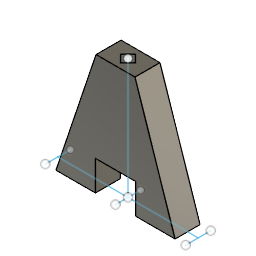
Leg (Autodesk Fusion 360 design; units mm, degrees)
part number: 2025-11-29-20-59-17-478
Autodesk Fusion 360 part; units mm, degrees
sketch "Sketch1" plane through (0, 0, 0) normal (0, 0, 1) x (1, 0, 0)
sketch "Sketch2" plane through (0, 0, 0) normal (0, 0, 1) x (1, 0, 0)
  circle A0 centre (0, 0) radius 100
  constraint coincident A0.centre origin
sketch "Sketch3" plane through (0, 0, 0) normal (0, 0, 1) x (1, 0, 0)
  circle A0 centre (0, -70) radius 17.5
  circle A1 centre (0, 70) radius 17.5
  dimension "d3" = 35
  dimension "d4" = 35
  measures "d3" diameter of A0
  measures "d4" diameter of A1
sketch "Sketch4" plane through (0, 0, 0) normal (0, 0, 1) x (1, 0, 0)
  circle A0 centre (0, -70) radius 5.25
  circle A1 centre (0, 70) radius 5.25
  dimension "d7" = 10.5
  dimension "d8" = 10.5
  measures "d7" diameter of A0
  measures "d8" diameter of A1
sketch "Sketch5" plane through (0, 0, 30) normal (0, 0, 1) x (-1, 0, 0)
  circle A0 centre (0, -70) radius 5.25
  circle A1 centre (0, 70) radius 5.25
  circle A2 centre (0, 0) radius 100
  circle A3 centre (0, 0) radius 50
  constraint coincident A2.centre A3.centre
sketch "Sketch6" plane through (0, 0, 0) normal (0, 0, 1) x (1, 0, 0)
  line L0 (125, -10) -> (90, -10)
  line L1 (90, -10) -> (90, 15)
  line L2 (90, 15) -> (125, 15)
  line L3 (125, 15) -> (125, -10)
  constraint horizontal L0
  constraint vertical L1
  constraint horizontal L2
  constraint vertical L3
sketch "Sketch7" plane through (0, 0, 15) normal (0, 0, 1) x (-1, 0, 0)
  circle A0 centre (0, 0) radius 50
sketch "Sketch17" plane through (0, 0, 0) normal (0, 0, 1) x (1, 0, 0)
  line L0 (-50, 25) -> (90, 25)
  line L1 (90, 25) -> (90, 0)
  line L2 (90, 0) -> (-50, 0)
  line L3 (-50, 0) -> (-50, 25)
  constraint horizontal L0
  constraint vertical L1
  constraint horizontal L2
  constraint vertical L3
extrude "Extrude19" add sketch "Sketch17" along normal blind 120
sketch "Sketch18" plane through (0, 0, 120) normal (0, 0, 1) x (-1, 0, 0)
  line L0 (50, 0) -> (-90, 0)
  line L1 (-90, 0) -> (-90, -25)
  line L2 (-90, -25) -> (50, -25)
  line L3 (50, -25) -> (50, 0)
  line L4 (50, 0) -> (50, -12.5)
  line L5 (50, -12.5) -> (-90, -12.5)
  line L6 (-20, -25) -> (-20, 0)
  line L7 (-12.9289, -12.5) -> (-20, -5.4289)
  line L8 (-20, -5.4289) -> (-27.0711, -12.5)
  line L9 (-27.0711, -12.5) -> (-20, -19.5711)
  line L10 (-20, -19.5711) -> (-12.9289, -12.5)
  line L11 (-12.9289, -12.5) -> (-27.0711, -12.5)
  line L12 (-20, -19.5711) -> (-20, -5.4289)
  constraint coincident L0.start L3.end
  constraint midpoint L3 L4.end
  constraint midpoint L1 L5.end
  constraint midpoint L2 L6.start
  constraint midpoint L0 L6.end
  constraint perpendicular L7 L8
  constraint perpendicular L8 L9
  constraint perpendicular L7 L10
  constraint perpendicular L11 L12
sketch "Sketch19" plane through (0, 0, 120) normal (0, 0, 1) x (-1, 0, 0)
sketch "Sketch20" plane through (0, 0, 0) normal (0, -1, 0) x (1, 0, 0)
sketch "Sketch21" plane through (0, 0, 120) normal (0, 0, 1) x (1, 0, 0)
  line L0 (90, 25, -120) -> (90, 0, -120)
  line L1 (-50, 25, -120) -> (-50, 0, -120)
  line L2 (20, 0, -120) -> (20, 25, -120)
  line L3 (-50, 12.5, -120) -> (90, 12.5, -120)
sketch "Sketch22" plane through (0, 0, 0) normal (0, 1, 0) x (1, 0, 0)
  line L0 (20, 0, 12.5) -> (20, -120, 12.5)
extrude "Extrude20" cut sketch "Sketch18" against normal blind 125 contours L5 L6 L7 L11 L12 | L5 L6 L8 L11 L12 | L5 L6 L10 L11 L12 | L5 L6 L9 L11 L12
sketch "Sketch23" plane through (0, 0, 0) normal (0, -1, 0) x (1, 0, 0)
  line L0 (-10, 120) -> (-50, 0)
  line L1 (-50, 0) -> (-50, 120)
  line L2 (-50, 120) -> (-10, 120)
  line L3 (90, 0) -> (50, 120)
  line L4 (50, 120) -> (90, 120)
  line L5 (90, 120) -> (90, 0)
  constraint vertical L1
  constraint perpendicular L1 L2
  constraint parallel L2 L4
  constraint perpendicular L4 L5
extrude "Extrude21" cut sketch "Sketch23" against normal blind 80
sketch "Sketch24" plane through (0, 0, 0) normal (0, 0, 1) x (1, 0, 0)
  line L0 (0, 25) -> (40, 25)
  line L1 (40, 25) -> (40, 0)
  line L2 (40, 0) -> (0, 0)
  line L3 (0, 0) -> (0, 25)
  constraint horizontal L0
  constraint vertical L1
  constraint horizontal L2
  constraint vertical L3
extrude "Extrude22" add 1 faces at (17.643, 17.214, 40) along direction (0.707107, -0.707107, 0) blind 10
sketch "Sketch25" plane through (0, 0, 0) normal (0, 0, 1) x (1, 0, 0)
  line L0 (20, 5.0754) -> (12.5754, 12.5)
  line L1 (12.5754, 12.5) -> (20, 19.9246)
  line L2 (20, 19.9246) -> (27.4246, 12.5)
  line L3 (27.4246, 12.5) -> (20, 5.0754)
  line L4 (20, 19.9246) -> (20, 5.0754)
  line L5 (27.4246, 12.5) -> (12.5754, 12.5)
  dimension "d52" = 10.5
  dimension "d53" = 10.5
  constraint perpendicular L0 L1
  constraint perpendicular L1 L2
  constraint perpendicular L0 L3
  measures "d52" distance of L0.start L0.end
  measures "d53" distance of L0.end L1.end
sketch "Sketch26" plane through (0, 0, 0) normal (0, 0, 1) x (1, 0, 0)
extrude "Extrude23" cut sketch "Sketch25" along normal blind 155
sketch "Sketch27" plane through (0, 0, 0) normal (0, 0, 1) x (1, 0, 0)
extrude "Extrude24" cut sketch "Sketch24" along normal blind 30
extrude "Extrude25" cut 1 faces at (-36.6667, 16.6667, 40) along direction (0.948683, 0, -0.316228) blind 10
extrude "Extrude26" cut 1 faces at (-6.8377, 8.3333, 118.9459) along direction (0.316228, 0, 0.948683) blind 30
extrude "Extrude27" cut 1 faces at (63.3333, 16.6667, 80) along direction (-0.948683, 0, -0.316228) blind 10
extrude "Extrude28" cut 1 faces at (43.6754, 8.3333, 117.8918) along direction (-0.316228, 0, 0.948683) blind 30
sketch "Sketch8" plane through (0, 12.5, 0) normal (0, 1, 0) x (-1, 0, 0)
  line L0 (-125, 0) -> (-90, 0)
  line L1 (-90, 0) -> (-90, 10)
  line L2 (-90, 10) -> (-125, 10)
  line L3 (-125, 10) -> (-125, 0)
  line L4 (-125, 0) -> (-100, 10)
  line L5 (-125, 10) -> (-125, 0)
  constraint coincident L0.start L3.end
  constraint coincident L2 L4.end
  constraint coincident L2.end L3.start
copy_body "CopyPasteBodies1" [suppressed]
move_body "Move2" [suppressed]
copy_body "CopyPasteBodies2" [suppressed]
move_body "Move3" [suppressed]
copy_body "CopyPasteBodies3" [suppressed]
combine "Combine1" [suppressed]
combine "Combine3" [suppressed]
combine "Combine5" [suppressed]
sketch "Sketch9" plane through (0, 0, 30) normal (0, 0, 1) x (-1, 0, 0)
  circle A0 centre (0, 0) radius 50
  circle A1 centre (0, -70) radius 5.25
  circle A2 centre (0, 70) radius 5.25
  circle A3 centre (0, 0) radius 100
  circle A4 centre (220, -250) radius 90
extrude "Extrude9" [suppressed]
sketch "Sketch10" plane through (0, 0, 30) normal (0, 0, 1) x (-1, 0, 0)
  circle A0 centre (0, 0) radius 50
  circle A1 centre (0, -70) radius 5.25
  circle A2 centre (0, 70) radius 5.25
  circle A3 centre (0, 0) radius 100
sketch "Sketch11" plane through (0, 0, 35) normal (0, 0, 1) x (-1, 0, 0)
  circle A0 centre (220, -250) radius 90
  circle A1 centre (290, -250) radius 5.25
  circle A2 centre (150, -250) radius 5.25
  dimension "d23" = 10.5
  dimension "d24" = 10.5
  measures "d23" diameter of A1
  measures "d24" diameter of A2
extrude "Extrude10" [suppressed]
move_body "Move5" [suppressed]
sketch "Sketch12" plane through (0, 0, 30) normal (0, 0, 1) x (-1, 0, 0)
  circle A0 centre (220, -250) radius 25
  dimension "d27" = 50
  measures "d27" diameter of A0
extrude "Extrude11" [suppressed]
sketch "Sketch13" plane through (0, 0, 0) normal (0, 0, 1) x (1, 0, 0)
extrude "Extrude12" [suppressed]
move_body "Move6" [suppressed]
move_body "Move7" [suppressed]
move_body "Move8" [suppressed]
sketch "Sketch14" plane through (0, 0, 5) normal (0, 0, 1) x (-1, 0, 0)
  circle A0 centre (0, -225) radius 25
  circle A1 centre (0, -295) radius 5.25
  circle A2 centre (0, -155) radius 5.25
  circle A3 centre (0, -225) radius 90
extrude "Extrude13" [suppressed]
sketch "Sketch15" plane through (0, 0, 0) normal (0, 0, 1) x (1, 0, 0)
  circle A0 centre (0, 0) radius 50
  constraint coincident A0.centre origin
extrude "Extrude14" [suppressed]
extrude "Extrude15" [suppressed]
sketch "Sketch16" plane through (0, 0, 0) normal (0, 0, 1) x (1, 0, 0)
  circle A0 centre (0, 0) radius 50
  constraint coincident A0.centre origin
extrude "Extrude16" [suppressed]
extrude "Extrude17" [suppressed]
